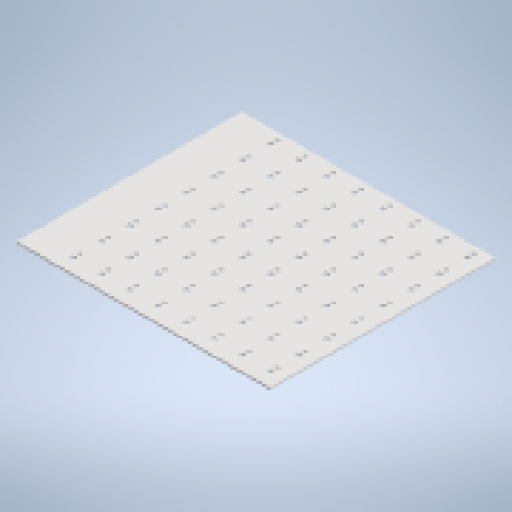
# Autodesk Inventor part: LED Holder
Saved by Autodesk Inventor 2025.2 (Build 292293000, 293)
## iProperties
Created: 2025-04-21
Part Number: LED Holder
Material: Generic
Document SubType Name: Modeling
Designer: powel
Density: 1 g/cm^3
Appearance: Default
Author: powel
Autodesk Inventor part; units mm, degrees
ref_plane "YZ Plane" through (0, 0, 0) normal (1, 0, 0) x (0, 1, 0)
ref_plane "XZ Plane" through (0, 0, 0) normal (0, 1, 0) x (-1, 0, 0)
ref_plane "XY Plane" through (0, 0, 0) normal (0, 0, 1) x (1, 0, 0)
sketch "Sketch1" plane through (0, 0, 0) normal (0, 1, 0) x (-1, 0, 0)
  line L0 (0, 0) -> (256, 0)
  line L1 (256, 0) -> (256, -256)
  line L2 (256, -256) -> (0, -256)
  line L3 (0, -256) -> (0, 0)
  line L4 (0, 0) -> (0, -32)
  line L5 (0, -32) -> (32, -32)
  line L6 (32, -32) -> (0, -32)
  line L7 (0, -32) -> (0, 0)
  line L8 (0, 0) -> (32, 0)
  line L9 (32, 0) -> (32, -32)
  line L10 (0, -32) -> (0, -64)
  line L11 (0, -64) -> (32, -64)
  line L12 (32, -64) -> (0, -64)
  line L13 (0, -64) -> (0, -32)
  line L14 (0, -32) -> (32, -32)
  line L15 (32, -32) -> (32, -64)
  line L16 (0, -64) -> (0, -96)
  line L17 (0, -96) -> (32, -96)
  line L18 (32, -96) -> (0, -96)
  line L19 (0, -96) -> (0, -64)
  line L20 (0, -64) -> (32, -64)
  line L21 (32, -64) -> (32, -96)
  line L22 (0, -96) -> (0, -128)
  line L23 (0, -128) -> (32, -128)
  line L24 (32, -128) -> (0, -128)
  line L25 (0, -128) -> (0, -96)
  line L26 (0, -96) -> (32, -96)
  line L27 (32, -96) -> (32, -128)
  line L28 (0, -128) -> (0, -160)
  line L29 (0, -160) -> (32, -160)
  line L30 (32, -160) -> (0, -160)
  line L31 (0, -160) -> (0, -128)
  line L32 (0, -128) -> (32, -128)
  line L33 (32, -128) -> (32, -160)
  line L34 (0, -160) -> (0, -192)
  line L35 (0, -192) -> (32, -192)
  line L36 (32, -192) -> (0, -192)
  line L37 (0, -192) -> (0, -160)
  line L38 (0, -160) -> (32, -160)
  line L39 (32, -160) -> (32, -192)
  line L40 (0, -192) -> (0, -224)
  line L41 (0, -224) -> (32, -224)
  line L42 (32, -224) -> (0, -224)
  line L43 (0, -224) -> (0, -192)
  line L44 (0, -192) -> (32, -192)
  line L45 (32, -192) -> (32, -224)
  line L46 (0, -224) -> (0, -256)
  line L47 (0, -256) -> (32, -256)
  line L48 (32, -256) -> (0, -256)
  line L49 (0, -256) -> (0, -224)
  line L50 (0, -224) -> (32, -224)
  line L51 (32, -224) -> (32, -256)
  line L52 (32, 0) -> (32, -32)
  line L53 (32, -32) -> (64, -32)
  line L54 (64, -32) -> (32, -32)
  line L55 (32, -32) -> (32, 0)
  line L56 (32, 0) -> (64, 0)
  line L57 (64, 0) -> (64, -32)
  line L58 (32, -32) -> (32, -64)
  line L59 (32, -64) -> (64, -64)
  line L60 (64, -64) -> (32, -64)
  line L61 (32, -64) -> (32, -32)
  line L62 (32, -32) -> (64, -32)
  line L63 (64, -32) -> (64, -64)
  line L64 (32, -64) -> (32, -96)
  line L65 (32, -96) -> (64, -96)
  line L66 (64, -96) -> (32, -96)
  line L67 (32, -96) -> (32, -64)
  line L68 (32, -64) -> (64, -64)
  line L69 (64, -64) -> (64, -96)
  line L70 (32, -96) -> (32, -128)
  line L71 (32, -128) -> (64, -128)
  line L72 (64, -128) -> (32, -128)
  line L73 (32, -128) -> (32, -96)
  line L74 (32, -96) -> (64, -96)
  line L75 (64, -96) -> (64, -128)
  line L76 (32, -128) -> (32, -160)
  line L77 (32, -160) -> (64, -160)
  line L78 (64, -160) -> (32, -160)
  line L79 (32, -160) -> (32, -128)
  line L80 (32, -128) -> (64, -128)
  line L81 (64, -128) -> (64, -160)
  line L82 (32, -160) -> (32, -192)
  line L83 (32, -192) -> (64, -192)
  line L84 (64, -192) -> (32, -192)
  line L85 (32, -192) -> (32, -160)
  line L86 (32, -160) -> (64, -160)
  line L87 (64, -160) -> (64, -192)
  line L88 (32, -192) -> (32, -224)
  line L89 (32, -224) -> (64, -224)
  line L90 (64, -224) -> (32, -224)
  line L91 (32, -224) -> (32, -192)
  line L92 (32, -192) -> (64, -192)
  line L93 (64, -192) -> (64, -224)
  line L94 (32, -224) -> (32, -256)
  line L95 (32, -256) -> (64, -256)
  line L96 (64, -256) -> (32, -256)
  line L97 (32, -256) -> (32, -224)
  line L98 (32, -224) -> (64, -224)
  line L99 (64, -224) -> (64, -256)
  line L100 (64, 0) -> (64, -32)
  line L101 (64, -32) -> (96, -32)
  line L102 (96, -32) -> (64, -32)
  line L103 (64, -32) -> (64, 0)
  line L104 (64, 0) -> (96, 0)
  line L105 (96, 0) -> (96, -32)
  line L106 (64, -32) -> (64, -64)
  line L107 (64, -64) -> (96, -64)
  line L108 (96, -64) -> (64, -64)
  line L109 (64, -64) -> (64, -32)
  line L110 (64, -32) -> (96, -32)
  line L111 (96, -32) -> (96, -64)
  line L112 (64, -64) -> (64, -96)
  line L113 (64, -96) -> (96, -96)
  line L114 (96, -96) -> (64, -96)
  line L115 (64, -96) -> (64, -64)
  line L116 (64, -64) -> (96, -64)
  line L117 (96, -64) -> (96, -96)
  line L118 (64, -96) -> (64, -128)
  line L119 (64, -128) -> (96, -128)
  line L120 (96, -128) -> (64, -128)
  line L121 (64, -128) -> (64, -96)
  line L122 (64, -96) -> (96, -96)
  line L123 (96, -96) -> (96, -128)
  line L124 (64, -128) -> (64, -160)
  line L125 (64, -160) -> (96, -160)
  line L126 (96, -160) -> (64, -160)
  line L127 (64, -160) -> (64, -128)
  line L128 (64, -128) -> (96, -128)
  line L129 (96, -128) -> (96, -160)
  line L130 (64, -160) -> (64, -192)
  line L131 (64, -192) -> (96, -192)
  line L132 (96, -192) -> (64, -192)
  line L133 (64, -192) -> (64, -160)
  line L134 (64, -160) -> (96, -160)
  line L135 (96, -160) -> (96, -192)
  line L136 (64, -192) -> (64, -224)
  line L137 (64, -224) -> (96, -224)
  line L138 (96, -224) -> (64, -224)
  line L139 (64, -224) -> (64, -192)
  line L140 (64, -192) -> (96, -192)
  line L141 (96, -192) -> (96, -224)
  line L142 (64, -224) -> (64, -256)
  line L143 (64, -256) -> (96, -256)
  line L144 (96, -256) -> (64, -256)
  line L145 (64, -256) -> (64, -224)
  line L146 (64, -224) -> (96, -224)
  line L147 (96, -224) -> (96, -256)
  line L148 (96, 0) -> (96, -32)
  line L149 (96, -32) -> (128, -32)
  line L150 (128, -32) -> (96, -32)
  line L151 (96, -32) -> (96, 0)
  line L152 (96, 0) -> (128, 0)
  line L153 (128, 0) -> (128, -32)
  line L154 (96, -32) -> (96, -64)
  line L155 (96, -64) -> (128, -64)
  line L156 (128, -64) -> (96, -64)
  line L157 (96, -64) -> (96, -32)
  line L158 (96, -32) -> (128, -32)
  line L159 (128, -32) -> (128, -64)
  line L160 (96, -64) -> (96, -96)
  line L161 (96, -96) -> (128, -96)
  line L162 (128, -96) -> (96, -96)
  line L163 (96, -96) -> (96, -64)
  line L164 (96, -64) -> (128, -64)
  line L165 (128, -64) -> (128, -96)
  line L166 (96, -96) -> (96, -128)
  line L167 (96, -128) -> (128, -128)
  line L168 (128, -128) -> (96, -128)
  line L169 (96, -128) -> (96, -96)
  line L170 (96, -96) -> (128, -96)
  line L171 (128, -96) -> (128, -128)
  line L172 (96, -128) -> (96, -160)
  line L173 (96, -160) -> (128, -160)
  line L174 (128, -160) -> (96, -160)
  line L175 (96, -160) -> (96, -128)
  line L176 (96, -128) -> (128, -128)
  line L177 (128, -128) -> (128, -160)
  line L178 (96, -160) -> (96, -192)
  line L179 (96, -192) -> (128, -192)
  line L180 (128, -192) -> (96, -192)
  line L181 (96, -192) -> (96, -160)
  line L182 (96, -160) -> (128, -160)
  line L183 (128, -160) -> (128, -192)
  line L184 (96, -192) -> (96, -224)
  line L185 (96, -224) -> (128, -224)
  line L186 (128, -224) -> (96, -224)
  line L187 (96, -224) -> (96, -192)
  line L188 (96, -192) -> (128, -192)
  line L189 (128, -192) -> (128, -224)
  line L190 (96, -224) -> (96, -256)
  line L191 (96, -256) -> (128, -256)
  line L192 (128, -256) -> (96, -256)
  line L193 (96, -256) -> (96, -224)
  line L194 (96, -224) -> (128, -224)
  line L195 (128, -224) -> (128, -256)
  line L196 (128, 0) -> (128, -32)
  line L197 (128, -32) -> (160, -32)
  line L198 (160, -32) -> (128, -32)
  line L199 (128, -32) -> (128, 0)
  line L200 (128, 0) -> (160, 0)
  line L201 (160, 0) -> (160, -32)
  line L202 (128, -32) -> (128, -64)
  line L203 (128, -64) -> (160, -64)
  line L204 (160, -64) -> (128, -64)
  line L205 (128, -64) -> (128, -32)
  line L206 (128, -32) -> (160, -32)
  line L207 (160, -32) -> (160, -64)
  line L208 (128, -64) -> (128, -96)
  line L209 (128, -96) -> (160, -96)
  line L210 (160, -96) -> (128, -96)
  line L211 (128, -96) -> (128, -64)
  line L212 (128, -64) -> (160, -64)
  line L213 (160, -64) -> (160, -96)
  line L214 (128, -96) -> (128, -128)
  line L215 (128, -128) -> (160, -128)
  line L216 (160, -128) -> (128, -128)
  line L217 (128, -128) -> (128, -96)
  line L218 (128, -96) -> (160, -96)
  line L219 (160, -96) -> (160, -128)
  line L220 (128, -128) -> (128, -160)
  line L221 (128, -160) -> (160, -160)
  line L222 (160, -160) -> (128, -160)
  line L223 (128, -160) -> (128, -128)
  line L224 (128, -128) -> (160, -128)
  line L225 (160, -128) -> (160, -160)
  line L226 (128, -160) -> (128, -192)
  line L227 (128, -192) -> (160, -192)
  line L228 (160, -192) -> (128, -192)
  line L229 (128, -192) -> (128, -160)
  line L230 (128, -160) -> (160, -160)
  line L231 (160, -160) -> (160, -192)
  line L232 (128, -192) -> (128, -224)
  line L233 (128, -224) -> (160, -224)
  line L234 (160, -224) -> (128, -224)
  line L235 (128, -224) -> (128, -192)
  line L236 (128, -192) -> (160, -192)
  line L237 (160, -192) -> (160, -224)
  line L238 (128, -224) -> (128, -256)
  line L239 (128, -256) -> (160, -256)
  line L240 (160, -256) -> (128, -256)
  line L241 (128, -256) -> (128, -224)
  line L242 (128, -224) -> (160, -224)
  line L243 (160, -224) -> (160, -256)
  line L244 (160, 0) -> (160, -32)
  line L245 (160, -32) -> (192, -32)
  line L246 (192, -32) -> (160, -32)
  line L247 (160, -32) -> (160, 0)
  line L248 (160, 0) -> (192, 0)
  line L249 (192, 0) -> (192, -32)
  line L250 (160, -32) -> (160, -64)
  line L251 (160, -64) -> (192, -64)
  line L252 (192, -64) -> (160, -64)
  line L253 (160, -64) -> (160, -32)
  line L254 (160, -32) -> (192, -32)
  line L255 (192, -32) -> (192, -64)
  line L256 (160, -64) -> (160, -96)
  line L257 (160, -96) -> (192, -96)
  line L258 (192, -96) -> (160, -96)
  line L259 (160, -96) -> (160, -64)
  line L260 (160, -64) -> (192, -64)
  line L261 (192, -64) -> (192, -96)
  line L262 (160, -96) -> (160, -128)
  line L263 (160, -128) -> (192, -128)
  line L264 (192, -128) -> (160, -128)
  line L265 (160, -128) -> (160, -96)
  line L266 (160, -96) -> (192, -96)
  line L267 (192, -96) -> (192, -128)
  line L268 (160, -128) -> (160, -160)
  line L269 (160, -160) -> (192, -160)
  line L270 (192, -160) -> (160, -160)
  line L271 (160, -160) -> (160, -128)
  line L272 (160, -128) -> (192, -128)
  line L273 (192, -128) -> (192, -160)
  line L274 (160, -160) -> (160, -192)
  line L275 (160, -192) -> (192, -192)
  line L276 (192, -192) -> (160, -192)
  line L277 (160, -192) -> (160, -160)
  line L278 (160, -160) -> (192, -160)
  line L279 (192, -160) -> (192, -192)
  line L280 (160, -192) -> (160, -224)
  line L281 (160, -224) -> (192, -224)
  line L282 (192, -224) -> (160, -224)
  line L283 (160, -224) -> (160, -192)
  line L284 (160, -192) -> (192, -192)
  line L285 (192, -192) -> (192, -224)
  line L286 (160, -224) -> (160, -256)
  line L287 (160, -256) -> (192, -256)
  line L288 (192, -256) -> (160, -256)
  line L289 (160, -256) -> (160, -224)
  line L290 (160, -224) -> (192, -224)
  line L291 (192, -224) -> (192, -256)
  line L292 (192, 0) -> (192, -32)
  line L293 (192, -32) -> (224, -32)
  line L294 (224, -32) -> (192, -32)
  line L295 (192, -32) -> (192, 0)
  line L296 (192, 0) -> (224, 0)
  line L297 (224, 0) -> (224, -32)
  line L298 (192, -32) -> (192, -64)
  line L299 (192, -64) -> (224, -64)
  line L300 (224, -64) -> (192, -64)
  line L301 (192, -64) -> (192, -32)
  line L302 (192, -32) -> (224, -32)
  line L303 (224, -32) -> (224, -64)
  line L304 (192, -64) -> (192, -96)
  line L305 (192, -96) -> (224, -96)
  line L306 (224, -96) -> (192, -96)
  line L307 (192, -96) -> (192, -64)
  line L308 (192, -64) -> (224, -64)
  line L309 (224, -64) -> (224, -96)
  line L310 (192, -96) -> (192, -128)
  line L311 (192, -128) -> (224, -128)
  line L312 (224, -128) -> (192, -128)
  line L313 (192, -128) -> (192, -96)
  line L314 (192, -96) -> (224, -96)
  line L315 (224, -96) -> (224, -128)
  line L316 (192, -128) -> (192, -160)
  line L317 (192, -160) -> (224, -160)
  line L318 (224, -160) -> (192, -160)
  line L319 (192, -160) -> (192, -128)
  line L320 (192, -128) -> (224, -128)
  line L321 (224, -128) -> (224, -160)
  line L322 (192, -160) -> (192, -192)
  line L323 (192, -192) -> (224, -192)
  line L324 (224, -192) -> (192, -192)
  line L325 (192, -192) -> (192, -160)
  line L326 (192, -160) -> (224, -160)
  line L327 (224, -160) -> (224, -192)
  line L328 (192, -192) -> (192, -224)
  line L329 (192, -224) -> (224, -224)
  line L330 (224, -224) -> (192, -224)
  line L331 (192, -224) -> (192, -192)
  line L332 (192, -192) -> (224, -192)
  line L333 (224, -192) -> (224, -224)
  line L334 (192, -224) -> (192, -256)
  line L335 (192, -256) -> (224, -256)
  line L336 (224, -256) -> (192, -256)
  line L337 (192, -256) -> (192, -224)
  line L338 (192, -224) -> (224, -224)
  line L339 (224, -224) -> (224, -256)
  line L340 (224, 0) -> (224, -32)
  line L341 (224, -32) -> (256, -32)
  line L342 (256, -32) -> (224, -32)
  line L343 (224, -32) -> (224, 0)
  line L344 (224, 0) -> (256, 0)
  line L345 (256, 0) -> (256, -32)
  line L346 (224, -32) -> (224, -64)
  line L347 (224, -64) -> (256, -64)
  line L348 (256, -64) -> (224, -64)
  line L349 (224, -64) -> (224, -32)
  line L350 (224, -32) -> (256, -32)
  line L351 (256, -32) -> (256, -64)
  line L352 (224, -64) -> (224, -96)
  line L353 (224, -96) -> (256, -96)
  line L354 (256, -96) -> (224, -96)
  line L355 (224, -96) -> (224, -64)
  line L356 (224, -64) -> (256, -64)
  line L357 (256, -64) -> (256, -96)
  line L358 (224, -96) -> (224, -128)
  line L359 (224, -128) -> (256, -128)
  line L360 (256, -128) -> (224, -128)
  line L361 (224, -128) -> (224, -96)
  line L362 (224, -96) -> (256, -96)
  line L363 (256, -96) -> (256, -128)
  line L364 (224, -128) -> (224, -160)
  line L365 (224, -160) -> (256, -160)
  line L366 (256, -160) -> (224, -160)
  line L367 (224, -160) -> (224, -128)
  line L368 (224, -128) -> (256, -128)
  line L369 (256, -128) -> (256, -160)
  line L370 (224, -160) -> (224, -192)
  line L371 (224, -192) -> (256, -192)
  line L372 (256, -192) -> (224, -192)
  line L373 (224, -192) -> (224, -160)
  line L374 (224, -160) -> (256, -160)
  line L375 (256, -160) -> (256, -192)
  line L376 (224, -192) -> (224, -224)
  line L377 (224, -224) -> (256, -224)
  line L378 (256, -224) -> (224, -224)
  line L379 (224, -224) -> (224, -192)
  line L380 (224, -192) -> (256, -192)
  line L381 (256, -192) -> (256, -224)
  line L382 (224, -224) -> (224, -256)
  line L383 (224, -256) -> (256, -256)
  line L384 (256, -256) -> (224, -256)
  line L385 (224, -256) -> (224, -224)
  line L386 (224, -224) -> (256, -224)
  line L387 (256, -224) -> (256, -256)
  line L388 (18.5, -18.5) -> (13.5, -18.5)
  line L389 (13.5, -18.5) -> (13.5, -13.5)
  line L390 (13.5, -13.5) -> (18.5, -13.5)
  line L391 (18.5, -13.5) -> (18.5, -18.5)
  circle A0 centre (16, -23.5) radius 2.5
  line L392 (13.5, -45.5) -> (18.5, -45.5)
  line L393 (13.5, -50.5) -> (13.5, -45.5)
  line L394 (18.5, -50.5) -> (13.5, -50.5)
  line L395 (18.5, -45.5) -> (18.5, -50.5)
  circle A1 centre (16, -55.5) radius 2.5
  line L396 (13.5, -77.5) -> (18.5, -77.5)
  line L397 (13.5, -82.5) -> (13.5, -77.5)
  line L398 (18.5, -82.5) -> (13.5, -82.5)
  line L399 (18.5, -77.5) -> (18.5, -82.5)
  circle A2 centre (16, -87.5) radius 2.5
  line L400 (13.5, -109.5) -> (18.5, -109.5)
  line L401 (13.5, -114.5) -> (13.5, -109.5)
  line L402 (18.5, -114.5) -> (13.5, -114.5)
  line L403 (18.5, -109.5) -> (18.5, -114.5)
  circle A3 centre (16, -119.5) radius 2.5
  line L404 (13.5, -141.5) -> (18.5, -141.5)
  line L405 (13.5, -146.5) -> (13.5, -141.5)
  line L406 (18.5, -146.5) -> (13.5, -146.5)
  line L407 (18.5, -141.5) -> (18.5, -146.5)
  circle A4 centre (16, -151.5) radius 2.5
  line L408 (13.5, -173.5) -> (18.5, -173.5)
  line L409 (13.5, -178.5) -> (13.5, -173.5)
  line L410 (18.5, -178.5) -> (13.5, -178.5)
  line L411 (18.5, -173.5) -> (18.5, -178.5)
  circle A5 centre (16, -183.5) radius 2.5
  line L412 (13.5, -205.5) -> (18.5, -205.5)
  line L413 (13.5, -210.5) -> (13.5, -205.5)
  line L414 (18.5, -210.5) -> (13.5, -210.5)
  line L415 (18.5, -205.5) -> (18.5, -210.5)
  circle A6 centre (16, -215.5) radius 2.5
  line L416 (13.5, -237.5) -> (18.5, -237.5)
  line L417 (13.5, -242.5) -> (13.5, -237.5)
  line L418 (18.5, -242.5) -> (13.5, -242.5)
  line L419 (18.5, -237.5) -> (18.5, -242.5)
  circle A7 centre (16, -247.5) radius 2.5
  line L420 (45.5, -13.5) -> (50.5, -13.5)
  line L421 (45.5, -18.5) -> (45.5, -13.5)
  line L422 (50.5, -18.5) -> (45.5, -18.5)
  line L423 (50.5, -13.5) -> (50.5, -18.5)
  circle A8 centre (48, -23.5) radius 2.5
  line L424 (45.5, -45.5) -> (50.5, -45.5)
  line L425 (45.5, -50.5) -> (45.5, -45.5)
  line L426 (50.5, -50.5) -> (45.5, -50.5)
  line L427 (50.5, -45.5) -> (50.5, -50.5)
  circle A9 centre (48, -55.5) radius 2.5
  line L428 (45.5, -77.5) -> (50.5, -77.5)
  line L429 (45.5, -82.5) -> (45.5, -77.5)
  line L430 (50.5, -82.5) -> (45.5, -82.5)
  line L431 (50.5, -77.5) -> (50.5, -82.5)
  circle A10 centre (48, -87.5) radius 2.5
  line L432 (45.5, -109.5) -> (50.5, -109.5)
  line L433 (45.5, -114.5) -> (45.5, -109.5)
  line L434 (50.5, -114.5) -> (45.5, -114.5)
  line L435 (50.5, -109.5) -> (50.5, -114.5)
  circle A11 centre (48, -119.5) radius 2.5
  line L436 (45.5, -141.5) -> (50.5, -141.5)
  line L437 (45.5, -146.5) -> (45.5, -141.5)
  line L438 (50.5, -146.5) -> (45.5, -146.5)
  line L439 (50.5, -141.5) -> (50.5, -146.5)
  circle A12 centre (48, -151.5) radius 2.5
  line L440 (45.5, -173.5) -> (50.5, -173.5)
  line L441 (45.5, -178.5) -> (45.5, -173.5)
  line L442 (50.5, -178.5) -> (45.5, -178.5)
  line L443 (50.5, -173.5) -> (50.5, -178.5)
  circle A13 centre (48, -183.5) radius 2.5
  line L444 (45.5, -205.5) -> (50.5, -205.5)
  line L445 (45.5, -210.5) -> (45.5, -205.5)
  line L446 (50.5, -210.5) -> (45.5, -210.5)
  line L447 (50.5, -205.5) -> (50.5, -210.5)
  circle A14 centre (48, -215.5) radius 2.5
  line L448 (45.5, -237.5) -> (50.5, -237.5)
  line L449 (45.5, -242.5) -> (45.5, -237.5)
  line L450 (50.5, -242.5) -> (45.5, -242.5)
  line L451 (50.5, -237.5) -> (50.5, -242.5)
  circle A15 centre (48, -247.5) radius 2.5
  line L452 (77.5, -13.5) -> (82.5, -13.5)
  line L453 (77.5, -18.5) -> (77.5, -13.5)
  line L454 (82.5, -18.5) -> (77.5, -18.5)
  line L455 (82.5, -13.5) -> (82.5, -18.5)
  circle A16 centre (80, -23.5) radius 2.5
  line L456 (77.5, -45.5) -> (82.5, -45.5)
  line L457 (77.5, -50.5) -> (77.5, -45.5)
  line L458 (82.5, -50.5) -> (77.5, -50.5)
  line L459 (82.5, -45.5) -> (82.5, -50.5)
  circle A17 centre (80, -55.5) radius 2.5
  line L460 (77.5, -77.5) -> (82.5, -77.5)
  line L461 (77.5, -82.5) -> (77.5, -77.5)
  line L462 (82.5, -82.5) -> (77.5, -82.5)
  line L463 (82.5, -77.5) -> (82.5, -82.5)
  circle A18 centre (80, -87.5) radius 2.5
  line L464 (77.5, -109.5) -> (82.5, -109.5)
  line L465 (77.5, -114.5) -> (77.5, -109.5)
  line L466 (82.5, -114.5) -> (77.5, -114.5)
  line L467 (82.5, -109.5) -> (82.5, -114.5)
  circle A19 centre (80, -119.5) radius 2.5
  line L468 (77.5, -141.5) -> (82.5, -141.5)
  line L469 (77.5, -146.5) -> (77.5, -141.5)
  line L470 (82.5, -146.5) -> (77.5, -146.5)
  line L471 (82.5, -141.5) -> (82.5, -146.5)
  circle A20 centre (80, -151.5) radius 2.5
  line L472 (77.5, -173.5) -> (82.5, -173.5)
  line L473 (77.5, -178.5) -> (77.5, -173.5)
  line L474 (82.5, -178.5) -> (77.5, -178.5)
  line L475 (82.5, -173.5) -> (82.5, -178.5)
  circle A21 centre (80, -183.5) radius 2.5
  line L476 (77.5, -205.5) -> (82.5, -205.5)
  line L477 (77.5, -210.5) -> (77.5, -205.5)
  line L478 (82.5, -210.5) -> (77.5, -210.5)
  line L479 (82.5, -205.5) -> (82.5, -210.5)
  circle A22 centre (80, -215.5) radius 2.5
  line L480 (77.5, -237.5) -> (82.5, -237.5)
  line L481 (77.5, -242.5) -> (77.5, -237.5)
  line L482 (82.5, -242.5) -> (77.5, -242.5)
  line L483 (82.5, -237.5) -> (82.5, -242.5)
  circle A23 centre (80, -247.5) radius 2.5
  line L484 (109.5, -13.5) -> (114.5, -13.5)
  line L485 (109.5, -18.5) -> (109.5, -13.5)
  line L486 (114.5, -18.5) -> (109.5, -18.5)
  line L487 (114.5, -13.5) -> (114.5, -18.5)
  circle A24 centre (112, -23.5) radius 2.5
  line L488 (109.5, -45.5) -> (114.5, -45.5)
  line L489 (109.5, -50.5) -> (109.5, -45.5)
  line L490 (114.5, -50.5) -> (109.5, -50.5)
  line L491 (114.5, -45.5) -> (114.5, -50.5)
  circle A25 centre (112, -55.5) radius 2.5
  line L492 (109.5, -77.5) -> (114.5, -77.5)
  line L493 (109.5, -82.5) -> (109.5, -77.5)
  line L494 (114.5, -82.5) -> (109.5, -82.5)
  line L495 (114.5, -77.5) -> (114.5, -82.5)
  circle A26 centre (112, -87.5) radius 2.5
  line L496 (109.5, -109.5) -> (114.5, -109.5)
  line L497 (109.5, -114.5) -> (109.5, -109.5)
  line L498 (114.5, -114.5) -> (109.5, -114.5)
  line L499 (114.5, -109.5) -> (114.5, -114.5)
  circle A27 centre (112, -119.5) radius 2.5
  line L500 (109.5, -141.5) -> (114.5, -141.5)
  line L501 (109.5, -146.5) -> (109.5, -141.5)
  line L502 (114.5, -146.5) -> (109.5, -146.5)
  line L503 (114.5, -141.5) -> (114.5, -146.5)
  circle A28 centre (112, -151.5) radius 2.5
  line L504 (109.5, -173.5) -> (114.5, -173.5)
  line L505 (109.5, -178.5) -> (109.5, -173.5)
  line L506 (114.5, -178.5) -> (109.5, -178.5)
  line L507 (114.5, -173.5) -> (114.5, -178.5)
  circle A29 centre (112, -183.5) radius 2.5
  line L508 (109.5, -205.5) -> (114.5, -205.5)
  line L509 (109.5, -210.5) -> (109.5, -205.5)
  line L510 (114.5, -210.5) -> (109.5, -210.5)
  line L511 (114.5, -205.5) -> (114.5, -210.5)
  circle A30 centre (112, -215.5) radius 2.5
  line L512 (109.5, -237.5) -> (114.5, -237.5)
  line L513 (109.5, -242.5) -> (109.5, -237.5)
  line L514 (114.5, -242.5) -> (109.5, -242.5)
  line L515 (114.5, -237.5) -> (114.5, -242.5)
  circle A31 centre (112, -247.5) radius 2.5
  line L516 (141.5, -13.5) -> (146.5, -13.5)
  line L517 (141.5, -18.5) -> (141.5, -13.5)
  line L518 (146.5, -18.5) -> (141.5, -18.5)
  line L519 (146.5, -13.5) -> (146.5, -18.5)
  circle A32 centre (144, -23.5) radius 2.5
  line L520 (141.5, -45.5) -> (146.5, -45.5)
  line L521 (141.5, -50.5) -> (141.5, -45.5)
  line L522 (146.5, -50.5) -> (141.5, -50.5)
  line L523 (146.5, -45.5) -> (146.5, -50.5)
  circle A33 centre (144, -55.5) radius 2.5
  line L524 (141.5, -77.5) -> (146.5, -77.5)
  line L525 (141.5, -82.5) -> (141.5, -77.5)
  line L526 (146.5, -82.5) -> (141.5, -82.5)
  line L527 (146.5, -77.5) -> (146.5, -82.5)
  circle A34 centre (144, -87.5) radius 2.5
  line L528 (141.5, -109.5) -> (146.5, -109.5)
  line L529 (141.5, -114.5) -> (141.5, -109.5)
  line L530 (146.5, -114.5) -> (141.5, -114.5)
  line L531 (146.5, -109.5) -> (146.5, -114.5)
  circle A35 centre (144, -119.5) radius 2.5
  line L532 (141.5, -141.5) -> (146.5, -141.5)
  line L533 (141.5, -146.5) -> (141.5, -141.5)
  line L534 (146.5, -146.5) -> (141.5, -146.5)
  line L535 (146.5, -141.5) -> (146.5, -146.5)
  circle A36 centre (144, -151.5) radius 2.5
  line L536 (141.5, -173.5) -> (146.5, -173.5)
  line L537 (141.5, -178.5) -> (141.5, -173.5)
  line L538 (146.5, -178.5) -> (141.5, -178.5)
  line L539 (146.5, -173.5) -> (146.5, -178.5)
  circle A37 centre (144, -183.5) radius 2.5
  line L540 (141.5, -205.5) -> (146.5, -205.5)
  line L541 (141.5, -210.5) -> (141.5, -205.5)
  line L542 (146.5, -210.5) -> (141.5, -210.5)
  line L543 (146.5, -205.5) -> (146.5, -210.5)
  circle A38 centre (144, -215.5) radius 2.5
  line L544 (141.5, -237.5) -> (146.5, -237.5)
  line L545 (141.5, -242.5) -> (141.5, -237.5)
  line L546 (146.5, -242.5) -> (141.5, -242.5)
  line L547 (146.5, -237.5) -> (146.5, -242.5)
  circle A39 centre (144, -247.5) radius 2.5
  line L548 (173.5, -13.5) -> (178.5, -13.5)
  line L549 (173.5, -18.5) -> (173.5, -13.5)
  line L550 (178.5, -18.5) -> (173.5, -18.5)
  line L551 (178.5, -13.5) -> (178.5, -18.5)
  circle A40 centre (176, -23.5) radius 2.5
  line L552 (173.5, -45.5) -> (178.5, -45.5)
  line L553 (173.5, -50.5) -> (173.5, -45.5)
  line L554 (178.5, -50.5) -> (173.5, -50.5)
  line L555 (178.5, -45.5) -> (178.5, -50.5)
  circle A41 centre (176, -55.5) radius 2.5
  line L556 (173.5, -77.5) -> (178.5, -77.5)
  line L557 (173.5, -82.5) -> (173.5, -77.5)
  line L558 (178.5, -82.5) -> (173.5, -82.5)
  line L559 (178.5, -77.5) -> (178.5, -82.5)
  circle A42 centre (176, -87.5) radius 2.5
  line L560 (173.5, -109.5) -> (178.5, -109.5)
  line L561 (173.5, -114.5) -> (173.5, -109.5)
  line L562 (178.5, -114.5) -> (173.5, -114.5)
  line L563 (178.5, -109.5) -> (178.5, -114.5)
  circle A43 centre (176, -119.5) radius 2.5
  line L564 (173.5, -141.5) -> (178.5, -141.5)
  line L565 (173.5, -146.5) -> (173.5, -141.5)
  line L566 (178.5, -146.5) -> (173.5, -146.5)
  line L567 (178.5, -141.5) -> (178.5, -146.5)
  circle A44 centre (176, -151.5) radius 2.5
  line L568 (173.5, -173.5) -> (178.5, -173.5)
  line L569 (173.5, -178.5) -> (173.5, -173.5)
  line L570 (178.5, -178.5) -> (173.5, -178.5)
  line L571 (178.5, -173.5) -> (178.5, -178.5)
  circle A45 centre (176, -183.5) radius 2.5
  line L572 (173.5, -205.5) -> (178.5, -205.5)
  line L573 (173.5, -210.5) -> (173.5, -205.5)
  line L574 (178.5, -210.5) -> (173.5, -210.5)
  line L575 (178.5, -205.5) -> (178.5, -210.5)
  circle A46 centre (176, -215.5) radius 2.5
  line L576 (173.5, -237.5) -> (178.5, -237.5)
  line L577 (173.5, -242.5) -> (173.5, -237.5)
  line L578 (178.5, -242.5) -> (173.5, -242.5)
  line L579 (178.5, -237.5) -> (178.5, -242.5)
  circle A47 centre (176, -247.5) radius 2.5
  line L580 (205.5, -13.5) -> (210.5, -13.5)
  line L581 (205.5, -18.5) -> (205.5, -13.5)
  line L582 (210.5, -18.5) -> (205.5, -18.5)
  line L583 (210.5, -13.5) -> (210.5, -18.5)
  circle A48 centre (208, -23.5) radius 2.5
  line L584 (205.5, -45.5) -> (210.5, -45.5)
  line L585 (205.5, -50.5) -> (205.5, -45.5)
  line L586 (210.5, -50.5) -> (205.5, -50.5)
  line L587 (210.5, -45.5) -> (210.5, -50.5)
  circle A49 centre (208, -55.5) radius 2.5
  line L588 (205.5, -77.5) -> (210.5, -77.5)
  line L589 (205.5, -82.5) -> (205.5, -77.5)
  line L590 (210.5, -82.5) -> (205.5, -82.5)
  line L591 (210.5, -77.5) -> (210.5, -82.5)
  circle A50 centre (208, -87.5) radius 2.5
  line L592 (205.5, -109.5) -> (210.5, -109.5)
  line L593 (205.5, -114.5) -> (205.5, -109.5)
  line L594 (210.5, -114.5) -> (205.5, -114.5)
  line L595 (210.5, -109.5) -> (210.5, -114.5)
  circle A51 centre (208, -119.5) radius 2.5
  line L596 (205.5, -141.5) -> (210.5, -141.5)
  line L597 (205.5, -146.5) -> (205.5, -141.5)
  line L598 (210.5, -146.5) -> (205.5, -146.5)
  line L599 (210.5, -141.5) -> (210.5, -146.5)
  circle A52 centre (208, -151.5) radius 2.5
  line L600 (205.5, -173.5) -> (210.5, -173.5)
  line L601 (205.5, -178.5) -> (205.5, -173.5)
  line L602 (210.5, -178.5) -> (205.5, -178.5)
  line L603 (210.5, -173.5) -> (210.5, -178.5)
  circle A53 centre (208, -183.5) radius 2.5
  line L604 (205.5, -205.5) -> (210.5, -205.5)
  line L605 (205.5, -210.5) -> (205.5, -205.5)
  line L606 (210.5, -210.5) -> (205.5, -210.5)
  line L607 (210.5, -205.5) -> (210.5, -210.5)
  circle A54 centre (208, -215.5) radius 2.5
  line L608 (205.5, -237.5) -> (210.5, -237.5)
  line L609 (205.5, -242.5) -> (205.5, -237.5)
  line L610 (210.5, -242.5) -> (205.5, -242.5)
  line L611 (210.5, -237.5) -> (210.5, -242.5)
  circle A55 centre (208, -247.5) radius 2.5
  line L612 (237.5, -13.5) -> (242.5, -13.5)
  line L613 (237.5, -18.5) -> (237.5, -13.5)
  line L614 (242.5, -18.5) -> (237.5, -18.5)
  line L615 (242.5, -13.5) -> (242.5, -18.5)
  circle A56 centre (240, -23.5) radius 2.5
  line L616 (237.5, -45.5) -> (242.5, -45.5)
  line L617 (237.5, -50.5) -> (237.5, -45.5)
  line L618 (242.5, -50.5) -> (237.5, -50.5)
  line L619 (242.5, -45.5) -> (242.5, -50.5)
  circle A57 centre (240, -55.5) radius 2.5
  line L620 (237.5, -77.5) -> (242.5, -77.5)
  line L621 (237.5, -82.5) -> (237.5, -77.5)
  line L622 (242.5, -82.5) -> (237.5, -82.5)
  line L623 (242.5, -77.5) -> (242.5, -82.5)
  circle A58 centre (240, -87.5) radius 2.5
  line L624 (237.5, -109.5) -> (242.5, -109.5)
  line L625 (237.5, -114.5) -> (237.5, -109.5)
  line L626 (242.5, -114.5) -> (237.5, -114.5)
  line L627 (242.5, -109.5) -> (242.5, -114.5)
  circle A59 centre (240, -119.5) radius 2.5
  line L628 (237.5, -141.5) -> (242.5, -141.5)
  line L629 (237.5, -146.5) -> (237.5, -141.5)
  line L630 (242.5, -146.5) -> (237.5, -146.5)
  line L631 (242.5, -141.5) -> (242.5, -146.5)
  circle A60 centre (240, -151.5) radius 2.5
  line L632 (237.5, -173.5) -> (242.5, -173.5)
  line L633 (237.5, -178.5) -> (237.5, -173.5)
  line L634 (242.5, -178.5) -> (237.5, -178.5)
  line L635 (242.5, -173.5) -> (242.5, -178.5)
  circle A61 centre (240, -183.5) radius 2.5
  line L636 (237.5, -205.5) -> (242.5, -205.5)
  line L637 (237.5, -210.5) -> (237.5, -205.5)
  line L638 (242.5, -210.5) -> (237.5, -210.5)
  line L639 (242.5, -205.5) -> (242.5, -210.5)
  circle A62 centre (240, -215.5) radius 2.5
  line L640 (237.5, -237.5) -> (242.5, -237.5)
  line L641 (237.5, -242.5) -> (237.5, -237.5)
  line L642 (242.5, -242.5) -> (237.5, -242.5)
  line L643 (242.5, -237.5) -> (242.5, -242.5)
  circle A63 centre (240, -247.5) radius 2.5
  line L644 (256, 0) -> (288, 0)
  line L645 (288, 0) -> (288, -256)
  line L646 (288, -256) -> (256, -256)
  line L647 (256, -256) -> (256, 0)
  line L648 (284.75, -94.44) -> (259.25, -94.44)
  line L649 (259.25, -94.44) -> (259.25, -144.64)
  line L650 (259.25, -144.64) -> (284.75, -144.64)
  line L651 (284.75, -144.64) -> (284.75, -94.44)
  line L652 (281.28, -114.36) -> (262.72, -114.36)
  line L653 (262.72, -114.36) -> (262.72, -141.64)
  line L654 (262.72, -141.64) -> (281.28, -141.64)
  line L655 (281.28, -141.64) -> (281.28, -114.36)
  point P0 (272, -144.64)
  dimension "d0" = 256
  dimension "d1" = 256
  dimension "d6" = 32
  dimension "d9" = 32
  dimension "d18" = 5
  dimension "d19" = 13.5
  dimension "d20" = 13.5
  dimension "d24" = 32
  dimension "d27" = 32
  dimension "d32" = 32
  dimension "d33" = 25.5
  dimension "d34" = 50.2
  dimension "d42" = 27.28
  dimension "d43" = 18.56
  dimension "d44" = 3
  dimension "d45" = 3.47
  constraints: 1312 end point, 64 centre point, 12 parallel, 8 horizontal, 7 perpendicular, 2 vertical, 1 midpoint, 1 point on line, 1323 other
  measures "d0" distance of L1.end L2.end
  measures "d1" distance of L0.end L1.end
  measures "d6" distance of L0.start L10.start
  measures "d9" distance of L0.start L52.start
  measures "d18" distance of L388.start L388.end
  measures "d19" distance between parallel lines of L0 L390
  measures "d20" distance between parallel lines of L3 L389
  measures "d24" distance of L389.end L392.start
  measures "d27" distance of L389.end L420.start
  measures "d32" distance of L645.end L646.end
  measures "d33" distance of L650.end L649.end
  measures "d34" distance of L649.end L648.end
  measures "d42" distance of L652.end L653.end
  measures "d43" distance of L652.start L652.end
  measures "d44" distance from line of point (272, -144.64) L654
  measures "d45" distance between parallel lines of L651 L655
extrude "Extrusion1" add sketch "Sketch1" along normal blind 2.3622 contours L0 L9 L5 L3 | L0 L57 L53 L9 | L5 L15 L11 L3 | L0 L105 L101 L57 | L53 L63 L59 L15 | L11 L21 L17 L3 | L0 L153 L149 L105 | L101 L111 L107 L63 | L59 L69 L65 L21 | L17 L27 L23 L3 | L0 L201 L197 L153 | L149 L159 L155 L111 | L107 L117 L113 L69 | L65 L75 L71 L27 | L23 L33 L29 L3 | L0 L249 L245 L201 | L197 L207 L203 L159 | L155 L165 L161 L117 | L113 L123 L119 L75 | L71 L81 L77 L33 | L29 L39 L35 L3 | L0 L297 L293 L249 | L245 L255 L251 L207 | L203 L213 L209 L165 | L161 L171 L167 L123 | L119 L129 L125 L81 | L77 L87 L83 L39 | L35 L45 L41 L3 | L0 L1 L341 L297 | L293 L303 L299 L255 | L251 L261 L257 L213 | L209 L219 L215 L171 | L167 L177 L173 L129 | L125 L135 L131 L87 | L83 L93 L89 L45 | L41 L51 L2 L3 | L644 L645 L646 L1 | L341 L1 L347 L303 | L299 L309 L305 L261 | L257 L267 L263 L219 | L215 L225 L221 L177 | L173 L183 L179 L135 | L131 L141 L137 L93 | L89 L99 L2 L51 | L347 L1 L353 L309 | L305 L315 L311 L267 | L263 L273 L269 L225 | L221 L231 L227 L183 | L179 L189 L185 L141 | L137 L147 L2 L99 | L353 L1 L359 L315 | L311 L321 L317 L273 | L269 L279 L275 L231 | L227 L237 L233 L189 | L185 L195 L2 L147 | L2 L339 L377 L1 | L359 L1 L365 L321 | L317 L327 L323 L279 | L275 L285 L281 L237 | L233 L243 L2 L195 | L377 L333 L371 L1 | L2 L291 L329 L339 | L365 L1 L371 L327 | L323 L333 L329 L285 | L281 L291 L2 L243 | L651 L650 L649 L648 | L655 L654 L653 L652
extrude "Extrusion2" add sketch "Sketch1" against normal blind 5.2 contours L651 L650 L649 L648
extrude "Extrusion3" add sketch "Sketch1" against normal blind 10.2 contours L655 L654 L653 L652
body "Solid1"
